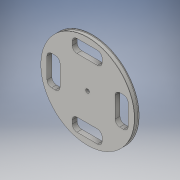
# Autodesk Inventor part: RTS  Wheel
Saved by Autodesk Inventor 2016 (Build 200138000, 138)
## iProperties
Created: 2016-10-11
Part Number: RTS  Wheel
Material: Generic
Document SubType Name: Modeling
Designer: sullir
Density: 1 g/cm^3
Appearance: Default
Author: sullir
Autodesk Inventor part; units mm, degrees
ref_plane "YZ Plane" through (0, 0, 0) normal (1, 0, 0) x (0, 1, 0)
ref_plane "XZ Plane" through (0, 0, 0) normal (0, 1, 0) x (-1, 0, 0)
ref_plane "XY Plane" through (0, 0, 0) normal (0, 0, 1) x (1, 0, 0)
sketch "Sketch1" plane through (0, 0, 0) normal (0, 0, 1) x (1, 0, 0)
  circle A0 centre (0, 0) radius 31.1101
  constraints: 1 centre point, 1 coincident
extrude "Extrusion1" add sketch "Sketch1" along normal blind 2.794
sketch "Sketch2" plane through (0, 0, 0) normal (0, 0, -1) x (-1, 0, 0)
  circle A0 centre (0, 0) radius 31.75
  dimension "d2" = 63.5
  constraints: 1 centre point, 1 coincident
  measures "d2" diameter of A0
extrude "Extrusion2" add sketch "Sketch2" along normal blind 0.254
sketch "Sketch3" plane through (0, 0, 2.794) normal (0, 0, 1) x (1, 0, 0)
  circle A0 centre (0, 0) radius 31.75
  dimension "d5" = 63.5
  constraints: 1 centre point, 1 coincident
  measures "d5" diameter of A0
extrude "Extrusion3" add sketch "Sketch3" along normal blind 0.254
sketch "Sketch4" plane through (0, 0, -0.254) normal (0, 0, -1) x (-1, 0, 0)
  arc A0 (-1.5256, 7.6067) -> (1.5256, 7.6067) centre (0, 8.5367) ccw
  line L0 (-1.5256, 7.6067) -> (-10.0877, 14.0155)
  arc A1 (-10.0877, 14.0155) -> (-14.0155, 10.0877) centre (-11.7691, 11.7691) ccw
  line L1 (-14.0155, 10.0877) -> (-7.6067, 1.5256)
  arc A2 (-7.6067, -1.5256) -> (-7.6067, 1.5256) centre (-8.5367, 0) ccw
  line L2 (-7.6067, -1.5256) -> (-14.0155, -10.0877)
  arc A3 (-14.0155, -10.0877) -> (-10.0877, -14.0155) centre (-11.7691, -11.7691) ccw
  line L3 (-10.0877, -14.0155) -> (-1.5256, -7.6067)
  arc A4 (1.5256, -7.6067) -> (-1.5256, -7.6067) centre (0, -8.5367) ccw
  line L4 (1.5256, -7.6067) -> (10.0877, -14.0155)
  arc A5 (10.0877, -14.0155) -> (14.0155, -10.0877) centre (11.7691, -11.7691) ccw
  line L5 (14.0155, -10.0877) -> (7.6067, -1.5256)
  arc A6 (7.6067, 1.5256) -> (7.6067, -1.5256) centre (8.5367, 0) ccw
  line L6 (7.6067, 1.5256) -> (14.0155, 10.0877)
  arc A7 (14.0155, 10.0877) -> (10.0877, 14.0155) centre (11.7691, 11.7691) ccw
  line L7 (10.0877, 14.0155) -> (1.5256, 7.6067)
  circle A8 centre (0, 0) radius 5.27
  circle A9 centre (-4.9144, 4.9144) radius 0.75
  circle A10 centre (-7.3893, 7.3893) radius 0.75
  circle A11 centre (-9.8641, 9.8641) radius 0.75
  circle A12 centre (-12.339, 12.339) radius 0.75
  circle A13 centre (-4.9144, -4.9144) radius 0.75
  circle A14 centre (-7.3893, -7.3893) radius 0.75
  circle A15 centre (-9.8641, -9.8641) radius 0.75
  circle A16 centre (-12.339, -12.339) radius 0.75
  circle A17 centre (4.9144, -4.9144) radius 0.75
  circle A18 centre (7.3893, -7.3893) radius 0.75
  circle A19 centre (9.8641, -9.8641) radius 0.75
  circle A20 centre (12.339, -12.339) radius 0.75
  circle A21 centre (4.9144, 4.9144) radius 0.75
  circle A22 centre (7.3893, 7.3893) radius 0.75
  circle A23 centre (9.8641, 9.8641) radius 0.75
  circle A24 centre (12.339, 12.339) radius 0.75
  constraints: 25 centre point, 16 end point, 16 point on circle
extrude "Extrusion4" cut sketch "Sketch4" against normal blind 1.3335 contours A0 L7 A7 L6 A6 L5 A5 L4 A4 L3 A3 L2 A2 L1 A1 L0 | A8 | A9 | A10 | A11 | A12 | A13 | A14 | A15 | A16 | A17 | A18 | A19 | A20 | A21 | A22 | A23 | A24
sketch "Sketch5" plane through (0, 0, -0.254) normal (0, 0, -1) x (-1, 0, 0)
  point P0 (0, 0)
hole "Hole1" at (0, 0, -0.254) direction (0, 0, 1) diameter 10.541 depth 1.5875
hole "Hole2" at (0.0046, 0.2595, 1.3335) direction (0, 0, 1) diameter 10.541 depth 0.254
sketch "Sketch6" plane through (0, 0, -0.254) normal (0, 0, -1) x (-1, 0, 0)
  line L0 (-6.735, 18.6967) -> (7.235, 18.6967)
  line L1 (10.41, 21.8717) -> (10.41, 24.4117)
  line L2 (7.235, 27.5867) -> (-6.735, 27.5867)
  line L3 (-9.91, 24.4117) -> (-9.91, 21.8717)
  line L4 (21.8717, 10.2323) -> (24.4117, 10.2323)
  line L5 (27.5867, 7.0573) -> (27.5867, -6.9127)
  line L6 (24.4117, -10.0877) -> (21.8717, -10.0877)
  line L7 (18.6967, -6.9127) -> (18.6967, 7.0573)
  arc A0 (7.6067, 1.5256) -> (7.6067, -1.5256) centre (8.5367, 0) ccw projected
  arc A1 (-1.5256, 7.6067) -> (1.5256, 7.6067) centre (0, 8.5367) ccw projected
  line L8 (-21.8717, -10.0877) -> (-24.4117, -10.0877)
  line L9 (-27.5867, -6.9127) -> (-27.5867, 7.0573)
  line L10 (-24.4117, 10.2323) -> (-21.8717, 10.2323)
  line L11 (-18.6967, 7.0573) -> (-18.6967, -6.9127)
  arc A2 (-7.6067, -1.5256) -> (-7.6067, 1.5256) centre (-8.5367, 0) ccw projected
  line L12 (7.235, -18.6967) -> (-6.735, -18.6967)
  line L13 (-9.91, -21.8717) -> (-9.91, -24.4117)
  line L14 (-6.735, -27.5867) -> (7.235, -27.5867)
  line L15 (10.41, -24.4117) -> (10.41, -21.8717)
  arc A3 (1.5256, -7.6067) -> (-1.5256, -7.6067) centre (0, -8.5367) ccw projected
  arc A4 (27.5867, 7.0573) -> (24.4117, 10.2323) centre (24.4117, 7.0573) ccw
  arc A5 (24.4117, -10.0877) -> (27.5867, -6.9127) centre (24.4117, -6.9127) ccw
  arc A6 (18.6967, -6.9127) -> (21.8717, -10.0877) centre (21.8717, -6.9127) ccw
  arc A7 (21.8717, 10.2323) -> (18.6967, 7.0573) centre (21.8717, 7.0573) ccw
  arc A8 (7.235, -27.5867) -> (10.41, -24.4117) centre (7.235, -24.4117) ccw
  arc A9 (-9.91, -24.4117) -> (-6.735, -27.5867) centre (-6.735, -24.4117) ccw
  arc A10 (-6.735, -18.6967) -> (-9.91, -21.8717) centre (-6.735, -21.8717) ccw
  arc A11 (10.41, -21.8717) -> (7.235, -18.6967) centre (7.235, -21.8717) ccw
  arc A12 (-6.735, 27.5867) -> (-9.91, 24.4117) centre (-6.735, 24.4117) ccw
  arc A13 (10.41, 24.4117) -> (7.235, 27.5867) centre (7.235, 24.4117) ccw
  arc A14 (-9.91, 21.8717) -> (-6.735, 18.6967) centre (-6.735, 21.8717) ccw
  arc A15 (7.235, 18.6967) -> (10.41, 21.8717) centre (7.235, 21.8717) ccw
  arc A16 (-27.5867, -6.9127) -> (-24.4117, -10.0877) centre (-24.4117, -6.9127) ccw
  arc A17 (-24.4117, 10.2323) -> (-27.5867, 7.0573) centre (-24.4117, 7.0573) ccw
  arc A18 (-21.8717, -10.0877) -> (-18.6967, -6.9127) centre (-21.8717, -6.9127) ccw
  arc A19 (-18.6967, 7.0573) -> (-21.8717, 10.2323) centre (-21.8717, 7.0573) ccw
  circle A20 centre (0, 0) radius 1.27
  point P0 (-9.91, 18.6967)
  point P1 (10.41, 27.5867)
  point P2 (10.41, 18.6967)
  point P3 (-9.91, 27.5867)
  point P4 (18.6967, 10.2323)
  point P5 (27.5867, -10.0877)
  point P6 (27.5867, 10.2323)
  point P7 (18.6967, -10.0877)
  point P8 (-18.6967, -10.0877)
  point P9 (-27.5867, 10.2323)
  point P10 (-27.5867, -10.0877)
  point P11 (-18.6967, 10.2323)
  point P12 (10.41, -18.6967)
  point P13 (-9.91, -27.5867)
  point P14 (-9.91, -18.6967)
  point P15 (10.41, -27.5867)
  dimension "d26" = 10.16
  dimension "d27" = 8.89
  dimension "d28" = 20.32
  dimension "d29" = 10.16
  dimension "d30" = 20.32
  dimension "d31" = 8.89
  dimension "d32" = 10.16
  dimension "d33" = 20.32
  dimension "d34" = 8.89
  dimension "d35" = 10.16
  dimension "d36" = 8.89
  dimension "d37" = 20.32
  dimension "d40" = 3.175
  dimension "d41" = 2.54
  constraints: 32 end point, 32 point on circle, 32 point on line, 32 tangent, 17 centre point, 15 equal radius, 8 parallel, 4 horizontal, 4 perpendicular, 1 coincident
  measures "d26" distance from line of A0.centre L7
  measures "d27" distance of point (27.587, -10.088) point (18.697, -10.088)
  measures "d28" distance between parallel lines of L6 L4
  measures "d29" distance from line of A1.centre L0
  measures "d30" distance of point (10.41, 27.587) point (-9.91, 27.587)
  measures "d31" distance of point (10.41, 18.697) point (10.41, 27.587)
  measures "d32" distance from line of A2.centre L11
  measures "d33" distance between parallel lines of L10 L8
  measures "d34" distance of point (-27.587, 10.232) point (-18.697, 10.232)
  measures "d35" distance from line of A3.centre L12
  measures "d36" distance of point (-9.91, -18.697) point (-9.91, -27.587)
  measures "d37" distance of point (-9.91, -27.587) point (10.41, -27.587)
  measures "d40" radius of A4
  measures "d41" diameter of A20
extrude "Extrusion5" cut sketch "Sketch6" against normal blind 38.1 contours A14 L3 A12 L2 A13 L1 A15 L0 | L4 A4 L5 A5 L6 A6 L7 A7 | L8 A16 L9 A17 L10 A19 L11 A18 | A11 L15 A8 L14 A9 L13 A10 L12
sketch "Sketch7" plane through (0.0046, 0.2595, 1.5875) normal (0, 0, -1) x (-1, 0, 0)
  circle A0 centre (0, 0) radius 1.27
  point P0 (0.0046, -0.2595)
  dimension "d42" = 2.54
  constraints: 1 centre point
  measures "d42" diameter of A0
extrude "Extrusion6" cut sketch "Sketch7" along normal mid plane 25.4
sketch "Sketch8" plane through (0.0046, 0.2595, 1.5875) normal (0, 0, -1) x (-1, 0, 0)
  circle A0 centre (0, 0) radius 5.4861
  point P0 (0.0046, -0.2595)
  constraints: 1 centre point
extrude "Extrusion7" cut sketch "Sketch8" along normal blind 1.5875
sketch "Sketch9" plane through (0.0046, 0.2595, 1.5875) normal (0, 0, -1) x (-1, 0, 0)
  circle A0 centre (0, 0) radius 5.715
  point P0 (0.0046, -0.2595)
  dimension "d47" = 11.43
  constraints: 1 centre point
  measures "d47" diameter of A0
extrude "Extrusion8" cut sketch "Sketch9" along normal blind 25.4
body "Solid1"
